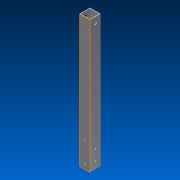
# Autodesk Inventor part: Front_Bar
Saved by Autodesk Inventor 2013 (Build 170138000, 138)
## iProperties
Created: 2013-07-13
Part Number: Front_Bar
Material: Aluminum 6061
Document SubType Name: Modeling
Designer: orange
Density: 1 g/cm^3
Author: orange
Autodesk Inventor part; units mm, degrees
ref_plane "YZ Plane" through (0, 0, 0) normal (1, 0, 0) x (0, 1, 0)
ref_plane "XZ Plane" through (0, 0, 0) normal (0, 1, 0) x (-1, 0, 0)
ref_plane "XY Plane" through (0, 0, 0) normal (0, 0, 1) x (1, 0, 0)
sketch "Sketch1" plane through (0, 0, 0) normal (0, 1, 0) x (-1, 0, 0)
  line L0 (0, 0) -> (25.4, 0)
  line L1 (25.4, 0) -> (25.4, 25.4)
  line L2 (25.4, 25.4) -> (0, 25.4)
  line L3 (0, 25.4) -> (0, 0)
  line L4 (1.651, 1.651) -> (23.749, 1.651)
  line L5 (23.749, 1.651) -> (23.749, 23.749)
  line L6 (23.749, 23.749) -> (1.651, 23.749)
  line L7 (1.651, 23.749) -> (1.651, 1.651)
  dimension "d0" = 25.4
  dimension "d1" = 25.4
  dimension "d2" = 1.651
  dimension "d3" = 1.651
  dimension "d4" = 1.651
  dimension "d5" = 1.651
  constraints: 16 end point, 4 parallel, 2 horizontal, 2 perpendicular
  measures "d0" distance of L2.end L0.start
  measures "d1" distance of L0.start L0.end
  measures "d2" distance between parallel lines of L7 L3
  measures "d3" distance between parallel lines of L6 L2
  measures "d4" distance between parallel lines of L1 L5
  measures "d5" distance between parallel lines of L0 L4
extrude "Extrusion1" add sketch "Sketch1" along normal blind 317.5
sketch "Sketch3" plane through (-25.4, 0, 25.4) normal (0, 0, 1) x (1, 0, 0)
  line L0 (0, 0) -> (25.4, 0) projected
  line L1 (25.4, 0) -> (25.4, 317.5) projected
  line L2 (0, 317.5) -> (25.4, 317.5) projected
  line L3 (0, 0) -> (0, 317.5) projected
sketch "Sketch4" plane through (-25.4, 0, 25.4) normal (0, 0, 1) x (1, 0, 0)
  line L0 (0, 0) -> (25.4, 0) projected
  line L1 (25.4, 0) -> (25.4, 317.5) projected
  point P0 (12.7, 12.7)
  point P1 (12.7, 63.5)
  dimension "d12" = 12.7
  dimension "d13" = 12.7
  dimension "d14" = 12.7
  dimension "d15" = 50.8
  measures "d12" distance from line of L1 point (12.7, 12.7)
  measures "d13" distance from line of L0 point (12.7, 12.7)
  measures "d14" distance from line of L1 point (12.7, 63.5)
  measures "d15" distance of point (12.7, 12.7) point (12.7, 63.5)
hole "Hole1" at (-12.7, 12.7, 25.4) direction (0, 0, -1) diameter 6.35 end through all
sketch "Sketch5" plane through (-25.4, 0, 25.4) normal (0, 0, 1) x (1, 0, 0)
  circle A0 centre (12.7, 12.7) radius 3.175 projected
  line L0 (25.4, 0) -> (25.4, 317.5) projected
  point P0 (12.7, 63.5)
  dimension "d23" = 12.7
  dimension "d24" = 50.8
  measures "d23" distance from line of L0 point (12.7, 63.5)
  measures "d24" distance of A0.centre point (12.7, 63.5)
hole "Hole2" at (-12.7, 63.5, 25.4) direction (0, 0, -1) diameter 6.35 end through all
sketch "Sketch6" plane through (0, 0, 25.4) normal (1, 0, 0) x (0, 0, -1)
  line L0 (0, 0) -> (25.4, 0) projected
  line L1 (25.4, 0) -> (25.4, 317.5) projected
  point P0 (12.7, 19.05)
  point P1 (12.7, 44.45)
  dimension "d32" = 12.7
  dimension "d33" = 12.7
  dimension "d34" = 19.05
  dimension "d35" = 25.4
  measures "d32" distance from line of L1 point (12.7, 19.05)
  measures "d33" distance from line of L1 point (12.7, 44.45)
  measures "d34" distance from line of L0 point (12.7, 19.05)
  measures "d35" distance of point (12.7, 19.05) point (12.7, 44.45)
hole "Hole3" at (0, 19.05, 12.7) at (0, 44.45, 12.7) direction (-1, 0, 0) diameter 6.35 end through all
sketch "Sketch7" plane through (0, 0, 25.4) normal (1, 0, 0) x (0, 0, -1)
  line L0 (0, 317.5) -> (25.4, 317.5) projected
  line L1 (0, 0) -> (0, 317.5) projected
  point P0 (12.7, 304.8)
  dimension "d43" = 12.7
  dimension "d44" = 12.7
  measures "d43" distance from line of L1 point (12.7, 304.8)
  measures "d44" distance from line of point (12.7, 304.8) L0
hole "Hole4" at (0, 304.8, 12.7) direction (-1, 0, 0) diameter 9.525 end through all
body "Solid1"
